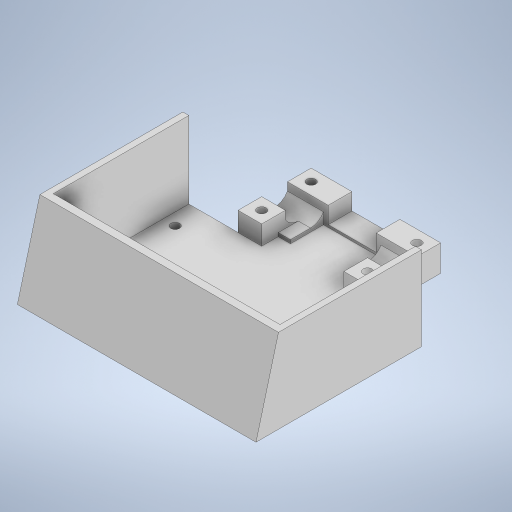
# Autodesk Inventor part: tělo estonsko
Saved by Autodesk Inventor 2024 (Build 280153000, 153)
## iProperties
Created: 2023-09-06
Part Number: tělo estonsko
Material: Všeobecné
Document SubType Name: Modeling
Designer: Simak
Density: 1 g/cm^3
Appearance: Výchozí
Author: Simak
Autodesk Inventor part; units mm, degrees
ref_plane "YZ Plane" through (0, 0, 0) normal (1, 0, 0) x (0, 1, 0)
ref_plane "XZ Plane" through (0, 0, 0) normal (0, 1, 0) x (-1, 0, 0)
ref_plane "XY Plane" through (0, 0, 0) normal (0, 0, 1) x (1, 0, 0)
sketch "Náčrt1" plane through (0, 0, 0) normal (0, 1, 0) x (-1, 0, 0)
  line L0 (49.75, -19.25) -> (49.75, 49.75)
  line L1 (49.75, 49.75) -> (-49.75, 49.75)
  line L2 (-49.75, 49.75) -> (-49.75, -19.25)
  line L3 (-49.75, -19.25) -> (-27.25, -19.25)
  line L4 (-27.25, -19.25) -> (-27.25, -49.75)
  line L5 (-27.25, -49.75) -> (26.75, -49.75)
  line L6 (26.75, -49.75) -> (26.75, -19.25)
  line L7 (26.75, -19.25) -> (49.75, -19.25)
  point P0 (0, 0)
  dimension "d0" = 30.5
  dimension "d1" = 99.5
  dimension "d2" = 22.5
  dimension "d3" = 99.5
  dimension "d4" = 54
  dimension "d5" = 49.75
  dimension "d6" = 49.75
  constraints: 16 end point, 6 perpendicular, 2 vertical, 1 parallel
  measures "d0" distance of L3.end L4.end
  measures "d1" distance of L0.end L1.end
  measures "d2" distance of L2.end L3.end
  measures "d3" distance between parallel lines of L1 L5
  measures "d4" distance of L4.end L5.end
  measures "d5" horizontal distance of L1.end point (0, 0)
  measures "d6" distance from line of point (0, 0) L1
extrude "Vysunutí1" add sketch "Náčrt1" along normal blind 3
sketch "Náčrt2" plane through (27.25, 0, -19.25) normal (1, 0, 0) x (0, 0, -1)
  line L0 (30.5, 3) -> (0, 3)
  line L1 (0, 3) -> (0, 11)
  line L2 (0, 11) -> (9.875, 11)
  line L3 (9.875, 11) -> (9.875, 7.646)
  arc A0 (9.875, 7.646) -> (20.625, 7.646) centre (15.25, 10.582835) ccw
  line L4 (20.625, 7.646) -> (20.625, 11)
  line L5 (20.625, 11) -> (30.5, 11)
  line L6 (30.5, 11) -> (30.5, 3)
  line L7 (0, 0) -> (30.5, 0)
  point P0 (-19.25, 0)
  dimension "d9" = 6.125
  dimension "d10" = 11
  dimension "d11" = 9.875
  dimension "d12" = 3.354
  constraints: 12 end point, 3 perpendicular, 2 equal length, 2 point on circle, 2 point on line, 1 centre point, 1 parallel, 1 vertical
  measures "d9" radius of A0
  measures "d10" distance between parallel lines of L5 L7
  measures "d11" distance of L4.end L5.end
  measures "d12" distance of L4.start L4.end
extrude "Vysunutí2" add sketch "Náčrt2" against normal up to surface (54 mm away)
sketch "Náčrt3" plane through (27.25, 3, -19.25) normal (0, 0, 1) x (1, 0, 0)
  line L0 (0, 8) -> (-54, 8) projected
  line L1 (-39, 8) -> (-39, 0)
  line L2 (-15, 8) -> (-15, 0)
  line L3 (-77, 0) -> (22.5, 0) projected
  line L4 (0, 8) -> (0, 0) projected
  line L5 (-54, 8) -> (-54, 0) projected
  line L6 (-15, 4) -> (0, 4)
  line L7 (-39, 4) -> (-54, 4)
  point P0 (-27.25, -3)
  dimension "d24" = 24
  constraints: 8 end point, 4 midpoint, 4 point on line, 2 vertical, 1 collinear
  measures "d24" distance between parallel lines of L1 L2
extrude "Vysunutí3" cut sketch "Náčrt3" against normal up to surface (20.625 mm away) contours L2 L3 L1 L0
sketch "Náčrt4" plane through (-26.75, 3, -19.25) normal (0, 0, 1) x (1, 0, 0)
  line L0 (0, 1.457835) -> (15, 1.457835)
  line L1 (39, 1.457835) -> (54, 1.457835)
  line L2 (9.875, 1.457835) -> (9.875, 8)
  line L3 (54, 8) -> (0, 8)
  line L4 (0, 8) -> (0, 0)
  line L5 (44.125, 8) -> (44.125, 1.457835)
  line L6 (54, 8) -> (54, 0)
  line L7 (15, 0) -> (15, 8)
  line L8 (39, 8) -> (39, 0)
  point P0 (26.75, -3)
  dimension "d20" = 9.875
  dimension "d21" = 9.875
  constraints: 4 end point, 4 point on line, 2 vertical
  measures "d20" distance between parallel lines of L4 L2
  measures "d21" distance between parallel lines of L6 L5
extrude "Vysunutí4" cut sketch "Náčrt4" against normal up to next contours L2 L3 L7 L0 | L8 L3 L5 L1
sketch "Náčrt5" plane through (-26.75, 3, -19.25) normal (0, 0, 1) x (1, 0, 0)
  line L0 (9.875, 1.457835) -> (9.875, 0)
  line L1 (15, 0) -> (0, 0)
  line L2 (44.125, 1.457835) -> (44.125, 0)
  line L3 (54, 0) -> (39, 0)
  line L4 (15, 1.457835) -> (9.875, 1.457835)
  line L5 (15, 0) -> (15, 1.457835)
  line L6 (-23, 0) -> (76.5, 0)
  line L7 (39, 1.457835) -> (39, 0)
  line L8 (44.125, 1.457835) -> (39, 1.457835)
  point P0 (26.75, -3)
  constraints: 4 end point, 2 coincident, 2 point on line, 1 parallel, 1 vertical
extrude "Vysunutí5" cut sketch "Náčrt5" against normal blind 6.875
sketch "Náčrt6" plane through (27.25, 7.646, -39.875) normal (0, 0, 1) x (1, 0, 0)
  line L0 (0, 3.354) -> (-54, 3.354) projected
  line L1 (-37, 3.354) -> (-37, -3.646)
  line L2 (-37, -3.646) -> (-17, -3.646)
  line L3 (-17, -3.646) -> (-17, 3.354)
  line L4 (-77, -4.646) -> (22.5, -4.646) projected
  line L5 (0, 3.354) -> (0, 0) projected
  line L6 (-17, -0.146) -> (0, -0.146) construction
  line L7 (-37, -0.146) -> (-54, -0.146) construction
  line L8 (-54, -7.646) -> (-54, 3.354) projected
  point P0 (-27.25, -7.646)
  dimension "d27" = 1
  dimension "d35" = 20
  constraints: 10 end point, 4 point on line, 2 horizontal, 2 midpoint, 2 perpendicular, 1 collinear, 1 vertical
  measures "d27" distance between parallel lines of L4 L2
  measures "d35" distance of L1.end L2.end
extrude "Vysunutí6" cut sketch "Náčrt6" against normal up to next
sketch "Náčrt7" plane through (-26.75, 11, -19.25) normal (0, 1, 0) x (1, 0, 0)
  circle A0 centre (4.9375, 4.9375) radius 1.85
  circle A1 centre (4.9375, 25.5625) radius 1.85
  circle A2 centre (49.0625, 25.5625) radius 1.85
  circle A3 centre (49.0625, 4.9375) radius 1.85
  line L0 (76.5, 0) -> (54, 0) projected
  line L1 (49.0625, 4.9375) -> (54, 0) construction
  line L2 (54, 0) -> (44.125, 0) projected
  line L3 (44.125, 0) -> (49.0625, 4.9375) construction
  line L4 (54, 9.875) -> (49.0625, 4.9375) construction
  line L5 (9.875, 0) -> (9.875, 6.875) projected
  line L6 (4.9375, 4.9375) -> (9.875, 0) construction
  line L7 (0, 30.5) -> (0, 0) projected
  line L8 (0, 0) -> (4.9375, 4.9375) construction
  line L9 (4.9375, 4.9375) -> (0, 9.875) construction
  line L10 (0, 20.625) -> (4.9375, 25.5625) construction
  line L11 (4.9375, 25.5625) -> (0, 30.5) construction
  line L12 (54, 0) -> (54, 30.5) projected
  line L13 (54, 20.625) -> (49.0625, 25.5625) construction
  line L14 (49.0625, 25.5625) -> (54, 30.5) construction
  point P0 (26.75, -19.25)
  dimension "d36" = 3.7
  constraints: 20 end point, 12 equal length, 4 centre point, 3 equal radius, 1 coincident
  measures "d36" diameter of A1
extrude "Vysunutí7" cut sketch "Náčrt7" against normal through all
sketch "Náčrt27" plane through (0, 0, 0) normal (0, -1, 0) x (1, 0, 0)
  circle A0 centre (22.3125, -44.8125) radius 1.85
  line L0 (19.4875, -43.181485) -> (22.3125, -41.550471)
  line L1 (22.3125, -41.550471) -> (25.1375, -43.181485)
  line L2 (25.1375, -43.181485) -> (25.1375, -46.443515)
  line L3 (25.1375, -46.443515) -> (22.3125, -48.074529)
  line L4 (22.3125, -48.074529) -> (19.4875, -46.443515)
  line L5 (19.4875, -46.443515) -> (19.4875, -43.181485)
  line L6 (19.4875, -25.818515) -> (19.4875, -22.556485)
  line L7 (19.4875, -22.556485) -> (22.3125, -20.925471)
  line L8 (22.3125, -20.925471) -> (25.1375, -22.556485)
  line L9 (25.1375, -22.556485) -> (25.1375, -25.818515)
  line L10 (25.1375, -25.818515) -> (22.3125, -27.449529)
  line L11 (22.3125, -27.449529) -> (19.4875, -25.818515)
  circle A1 centre (-21.8125, -24.1875) radius 1.85
  line L12 (-18.9875, -25.818515) -> (-21.8125, -27.449529)
  line L13 (-21.8125, -27.449529) -> (-24.6375, -25.818515)
  line L14 (-24.6375, -25.818515) -> (-24.6375, -22.556485)
  line L15 (-24.6375, -22.556485) -> (-21.8125, -20.925471)
  line L16 (-21.8125, -20.925471) -> (-18.9875, -22.556485)
  line L17 (-18.9875, -22.556485) -> (-18.9875, -25.818515)
  circle A2 centre (-21.8125, -44.8125) radius 1.85
  line L18 (-18.9875, -46.443515) -> (-21.8125, -48.074529)
  line L19 (-21.8125, -48.074529) -> (-24.6375, -46.443515)
  line L20 (-24.6375, -46.443515) -> (-24.6375, -43.181485)
  line L21 (-24.6375, -43.181485) -> (-21.8125, -41.550471)
  line L22 (-21.8125, -41.550471) -> (-18.9875, -43.181485)
  line L23 (-18.9875, -43.181485) -> (-18.9875, -46.443515)
  point P0 (0, 0)
  point P1 (22.3125, -24.1875)
  dimension "d179" = 5.65
  constraints: 48 end point, 4 vertical, 3 coincident, 3 equal length, 1 horizontal alignment, 1 vertical alignment, 52 other
  measures "d179" distance between parallel lines of L2 L5
extrude "Vysunutí30" cut sketch "Náčrt27" against normal blind 7 contours A0 | L0 L1 L2 L3 L4 L5 | L6 L7 L8 L9 L10 L11 | A1 | L12 L13 L14 L15 L16 L17 | A2 | L18 L19 L20 L21 L22 L23
chamfer "Zkosení2" distance 1 angle 45 4 edges at (20.4625, 7, -44.8125) (20.4625, 7, -24.1875) (-23.6625, 7, -24.1875) (-23.6625, 7, -44.8125)
sketch "Náčrt28" plane through (0, 3, 0) normal (0, 1, 0) x (1, 0, 0)
  circle A0 centre (-42.25, 8.5) radius 1.85
  circle A1 centre (42.25, 8.5) radius 1.85
  circle A2 centre (42.25, -29) radius 1.85
  circle A3 centre (-42.25, -29) radius 1.85
  line L0 (-42.25, 8.5) -> (-49.75, 8.5) construction
  line L1 (-49.75, 19.25) -> (-49.75, -49.75) projected
  line L2 (42.25, 8.5) -> (49.75, 8.5) construction
  line L3 (49.75, -49.75) -> (49.75, 19.25) projected
  line L4 (-49.75, -49.75) -> (49.75, -49.75) projected
  point P0 (0, 0)
  dimension "d185" = 3.7
  dimension "d186" = 84.5
  dimension "d187" = 37.5
  dimension "d195" = 20.75
  constraints: 4 centre point, 4 end point, 3 equal radius, 3 point on line, 2 horizontal alignment, 2 vertical alignment, 1 collinear, 1 horizontal
  measures "d185" diameter of A0
  measures "d186" distance of L2.start L0.start
  measures "d187" distance of A3.centre L0.start
  measures "d195" distance from line of L4 A3.centre
sketch "Náčrt29" plane through (49.75, 0, 49.75) normal (1, 0, 0) x (0, 0, -1)
  line L0 (0, 0) -> (69, 0)
  line L1 (0, 0) -> (9.378222, 35)
  line L2 (9.378222, 35) -> (12.48405, 35)
  line L3 (12.48405, 35) -> (3.909676, 3)
  line L4 (0, 3) -> (69, 3)
  line L5 (0, 0) -> (0, 3)
  point P0 (49.75, 0)
  point P1 (0.803848, 3)
  dimension "d188" = 75
  dimension "d189" = 35
  dimension "d190" = 3
  constraints: 6 end point, 1 horizontal, 1 parallel, 1 point on line
  measures "d188" angle of L0 L1
  measures "d189" distance between parallel lines of L0 L2
  measures "d190" distance between parallel lines of L1 L3
extrude "Vysunutí31" add sketch "Náčrt29" against normal up to surface (99.5 mm away) contours L1 L2 L3 L4
extrude "Vysunutí32" cut sketch "Náčrt29" against normal through all contours L5 L4 L1
extrude "Vysunutí33" cut sketch "Náčrt28" against normal up to next
sketch "Náčrt31" plane through (0, 3, 0) normal (0, 1, 0) x (1, 0, 0)
  line L0 (37.136, -36.833) -> (45.136, -36.833)
  line L1 (45.136, -36.833) -> (45.136, -44.833)
  line L2 (45.136, -44.833) -> (37.136, -44.833)
  line L3 (37.136, -44.833) -> (37.136, -36.833)
  line L4 (-4, -36.833) -> (4, -36.833)
  line L5 (4, -36.833) -> (4, -44.833)
  line L6 (4, -44.833) -> (-4, -44.833)
  line L7 (-4, -44.833) -> (-4, -36.833)
  line L8 (-45.463, -36.833) -> (-37.463, -36.833)
  line L9 (-37.463, -36.833) -> (-37.463, -44.833)
  line L10 (-37.463, -44.833) -> (-45.463, -44.833)
  line L11 (-45.463, -44.833) -> (-45.463, -36.833)
  line L12 (49.75, -45.840324) -> (49.75, 19.25)
  line L13 (-49.75, 19.25) -> (-49.75, -45.840324)
  line L14 (-49.75, -49.75) -> (49.75, -49.75)
  point P0 (0, 0)
  point P1 (0, -36.833)
  dimension "d198" = 8
  dimension "d199" = 4.614
  dimension "d200" = 4.287
  dimension "d201" = 4.917
  constraints: 24 end point, 6 parallel, 5 equal length, 3 horizontal, 3 perpendicular, 2 horizontal alignment, 1 midpoint, 1 point on line, 1 vertical alignment
  measures "d198" distance between parallel lines of L2 L0
  measures "d199" distance between parallel lines of L12 L1
  measures "d200" distance between parallel lines of L13 L11
  measures "d201" distance from line of L14 L5.end
extrude "Vysunutí34" cut sketch "Náčrt31" against normal up to next
sketch "Náčrt32" plane through (-26.75, 0, -19.25) normal (0, 0, -1) x (-1, 0, 0)
  line L0 (0, 0) -> (23, 0) projected
  line L1 (23, 0) -> (20.5, 0)
  line L2 (20.5, 0) -> (20.5, 35)
  line L3 (20.5, 35) -> (23, 35)
  line L4 (23, 35) -> (23, 0)
  line L5 (-76.5, 0) -> (-74, 0)
  line L6 (-74, 0) -> (-74, 35)
  line L7 (-74, 35) -> (-76.5, 35)
  line L8 (-76.5, 35) -> (-76.5, 0)
  line L9 (-76.5, 35) -> (23, 35) projected
  point P0 (-26.75, 0)
  dimension "d204" = 2.5
  constraints: 16 end point, 4 parallel, 2 horizontal, 2 perpendicular, 1 collinear, 1 point on line
  measures "d204" distance between parallel lines of L2 L4
extrude "Vysunutí35" add sketch "Náčrt32" against normal up to next
